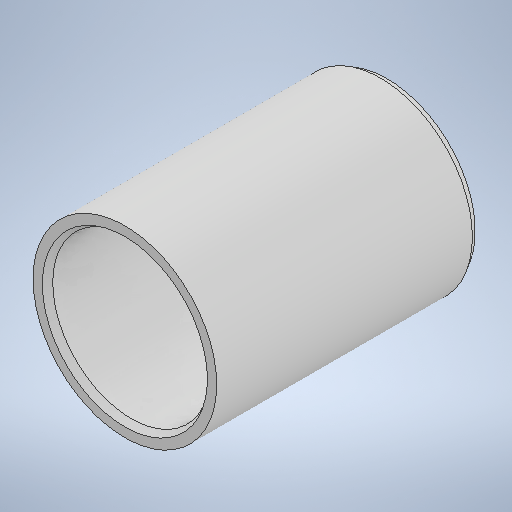
# Autodesk Inventor part: 47-02-004
Saved by Autodesk Inventor 2025.2 (Build 292293000, 293)
## iProperties
Created: 2025-01-09
Part Number: 47-02-004
Material: Generic
Document SubType Name: Modeling
Designer: Zvonko.Gabric
Density: 1 g/cm^3
Appearance: Default
Author: Zvonko.Gabric
Autodesk Inventor part; units mm, degrees
ref_plane "YZ Plane" through (0, 0, 0) normal (1, 0, 0) x (0, 1, 0)
ref_plane "XZ Plane" through (0, 0, 0) normal (0, 1, 0) x (-1, 0, 0)
ref_plane "XY Plane" through (0, 0, 0) normal (0, 0, 1) x (1, 0, 0)
sketch "Sketch1" plane through (0, 0, 0) normal (0, 1, 0) x (-1, 0, 0)
  line L0 (0, 0) -> (0, -20) construction
  line L1 (6.7115, -20) -> (7, -19.5)
  line L2 (7, -19.5) -> (7, 0)
  line L3 (7, 0) -> (6.2885, 0)
  line L4 (6.2885, 0) -> (6, -0.5)
  line L5 (6, -0.5) -> (6, -20)
  line L6 (6.7115, -20) -> (6, -20)
  dimension "d0" = 20
  dimension "d2" = 6
  dimension "d3" = 6.7115
  dimension "d4" = 0.5
  dimension "d5" = 7
  dimension "d6" = 6.2885
  constraints: 14 end point, 2 parallel, 1 horizontal, 1 perpendicular, 1 vertical
  measures "d0" distance of L0.start L0.end
  measures "d2" distance between parallel lines of L0 L5
  measures "d3" distance from line of L1.start L0
  measures "d4" vertical distance of L1.start L1.end
  measures "d5" distance between parallel lines of L0 L2
  measures "d6" distance from line of L0 L3.end
revolve "Revolution1" add sketch "Sketch1" angle 360 about axis through (0, 0, 0) along (0, 0, -1)
body "Solid1"
